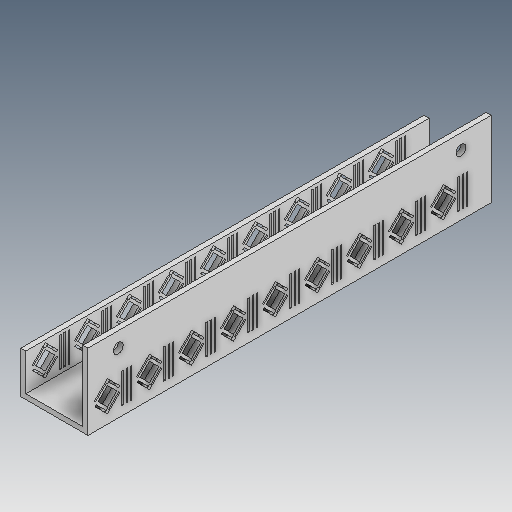
# Autodesk Inventor part: cable_basket
Saved by Autodesk Inventor 2027 (Build 310192060, 192F)
## iProperties
Created: 2026-07-28
Part Number: cable_basket
Material: Generic
Document SubType Name: Modeling
Designer: prest
Density: 1 g/cm^3
Appearance: Default
Author: prest
Autodesk Inventor part; units mm, degrees
ref_plane "YZ Plane" through (0, 0, 0) normal (1, 0, 0) x (0, 1, 0)
ref_plane "XZ Plane" through (0, 0, 0) normal (0, 1, 0) x (-1, 0, 0)
ref_plane "XY Plane" through (0, 0, 0) normal (0, 0, 1) x (1, 0, 0)
sketch "Sketch1" plane through (0, 0, 0) normal (0, 1, 0) x (-1, 0, 0)
  line L0 (65.1379, 125.1379) -> (25.1379, 125.1379)
  line L1 (25.1379, 125.1379) -> (25.1379, -114.8621)
  line L2 (25.1379, -114.8621) -> (65.1379, -114.8621)
  line L3 (65.1379, -114.8621) -> (65.1379, 125.1379)
  point P0 (0, 0)
  dimension "d0" = 240
  dimension "d1" = 40
  constraints: 8 end point, 2 parallel, 1 horizontal, 1 perpendicular
  measures "d0" distance of L2.end L0.start
  measures "d1" distance of L0.start L0.end
extrude "Extrusion1" add sketch "Sketch1" along normal blind 25
sketch "Sketch2" plane through (-65.1379, 0, 125.1379) normal (0, 0, 1) x (1, 0, 0)
  line L0 (0, 0) -> (0, 25) projected
  line L1 (0, 0) -> (40, 0) projected
  line L2 (40, 0) -> (40, 25) projected
  line L3 (3, 25) -> (3, 3)
  line L4 (3, 3) -> (37, 3)
  line L5 (37, 3) -> (37, 25)
  line L6 (3, 25) -> (37, 25)
  point P0 (65.1379, 0)
  dimension "d4" = 3
  constraints: 8 end point, 1 perpendicular, 2 other
  measures "d4" distance between parallel lines of L0 L3
extrude "Extrusion2" cut sketch "Sketch2" against normal through all
sketch "Sketch3" plane through (-65.1379, 0, -114.8621) normal (-1, 0, 0) x (0, 0, 1)
  line L0 (240, 3) -> (0, 3) projected
  line L1 (219.8357, 5.3002) -> (219.8357, 23)
  line L2 (219.8357, 23) -> (218.8357, 23)
  line L3 (218.8357, 23) -> (218.8357, 5.3002)
  line L4 (217.3357, 23) -> (216.3357, 23)
  line L5 (216.3357, 23) -> (216.3357, 5.3002)
  line L6 (217.3357, 5.3002) -> (217.3357, 23)
  line L7 (240, 0) -> (240, 25) projected
  line L8 (0, 25) -> (240, 25) projected
  line L9 (213.8357, 23) -> (214.8357, 23)
  line L10 (214.8357, 23) -> (214.8357, 5.3002)
  line L11 (213.8357, 5.3002) -> (213.8357, 23)
  line L12 (222.8357, 14.4178) -> (228.4178, 8.8357)
  line L13 (228.4178, 8.8357) -> (234, 14.4178)
  line L14 (234, 14.4178) -> (228.4178, 20)
  line L15 (228.4178, 20) -> (222.8357, 14.4178)
  line L16 (221.775, 15.4785) -> (227.3572, 21.0607)
  line L17 (229.4785, 21.0607) -> (235.4217, 15.1174)
  line L18 (235.0607, 13.3572) -> (229.4785, 7.775)
  line L19 (227.3572, 7.775) -> (221.775, 13.3572)
  line L20 (221.0679, 16.1856) -> (226.6501, 21.7678)
  line L21 (230.144, 21.8094) -> (236.1288, 15.8245)
  line L22 (226.6501, 7.0679) -> (221.0679, 12.6501)
  line L23 (235.7678, 12.6501) -> (230.1856, 7.0679)
  line L24 (221.0679, 16.1856) -> (221.775, 15.4785)
  line L25 (226.6501, 21.7678) -> (227.3572, 21.0607)
  line L26 (230.144, 21.8094) -> (229.4785, 21.0607)
  line L27 (236.1288, 15.8245) -> (235.4217, 15.1174)
  line L28 (235.0607, 13.3572) -> (235.7678, 12.6501)
  line L29 (226.6501, 7.0679) -> (227.3572, 7.775)
  line L30 (229.4785, 7.775) -> (230.1856, 7.0679)
  line L31 (221.0679, 12.6501) -> (221.775, 13.3572)
  line L32 (227.0036, 6.7144) -> (228.4178, 8.1286)
  line L33 (228.4178, 8.1286) -> (229.8321, 6.7144)
  line L34 (229.8321, 6.7144) -> (228.4178, 5.3002)
  line L35 (228.4178, 5.3002) -> (227.0036, 6.7144)
  line L36 (228.4178, 20.7071) -> (229.8321, 22.1213)
  line L37 (229.8321, 22.1213) -> (228.4178, 23.5355)
  line L38 (228.4178, 23.5355) -> (227.0036, 22.1213)
  line L39 (227.0036, 22.1213) -> (228.4178, 20.7071)
  line L40 (213.8357, 5.3002) -> (214.8357, 5.3002)
  line L41 (216.3357, 5.3002) -> (217.3357, 5.3002)
  line L42 (218.8357, 5.3002) -> (219.8357, 5.3002)
  line L43 (228.4178, 20) -> (228.4178, 8.8357) construction
  line L44 (222.8357, 14.4178) -> (234, 14.4178) construction
  point P0 (114.8621, 0)
  point P1 (216.8357, 23)
  point P2 (219.3357, 23)
  point P3 (214.3357, 23)
  point P4 (219.3357, 5.3002)
  dimension "d9" = 1
  dimension "d10" = 1
  dimension "d11" = 1.5
  dimension "d13" = 2
  dimension "d15" = 1
  dimension "d16" = 1.5
  dimension "d17" = 5
  dimension "d20" = 3
  dimension "d21" = 1.5
  dimension "d22" = 1.5
  dimension "d23" = 1
  dimension "d24" = 1
  dimension "d25" = 1
  dimension "d26" = 1
  dimension "d27" = 6
  dimension "d29" = 1.5
  dimension "d30" = 5.5822
  dimension "d31" = 0.5
  constraints: 84 end point, 24 perpendicular, 11 collinear, 6 horizontal, 5 vertical alignment, 4 horizontal alignment, 4 midpoint, 4 parallel, 2 point on line, 2 vertical
  measures "d9" distance of L1.end L2.end
  measures "d10" distance of L4.start L4.end
  measures "d11" distance between parallel lines of L3 L6
  measures "d13" distance from line of L8 point (216.836, 23)
  measures "d15" distance of L9.end L9.start
  measures "d16" distance of L4.end L9.end
  measures "d17" distance from line of L8 L14.end
  measures "d20" distance from line of L12.start L1
  measures "d21" distance between parallel lines of L15 L16
  measures "d22" distance between parallel lines of L17 L14
  measures "d23" distance between parallel lines of L16 L20
  measures "d24" distance between parallel lines of L17 L21
  measures "d25" distance between parallel lines of L19 L22
  measures "d26" distance between parallel lines of L18 L23
  measures "d27" distance from line of L7 L13.end
  measures "d29" distance between parallel lines of L12 L19
  measures "d30" horizontal distance of L12.end L13.end
  measures "d31" distance between parallel lines of L39 L25
extrude "Extrusion3" cut sketch "Sketch3" against normal through all
pattern_linear "Rectangular Pattern1" count 9 spacing 25 along (0, 0, -1) of "Extrusion3"
move faces "Move1" translate (0, 20, 0) faces at (-27.1379, 25, -34.8621)
sketch "Sketch5" plane through (-25.1379, 0, 125.1379) normal (1, 0, 0) x (0, 0, -1)
  line L0 (0, 0) -> (0, 45) projected
  line L1 (240, 3) -> (240, 45) projected
  line L2 (0, 45) -> (240, 45) projected
  point P0 (125.1379, 0)
  point P1 (18, 36)
  point P2 (222, 36)
  dimension "d40" = 204
  dimension "d41" = 18
  dimension "d43" = 9
  constraints: 1 horizontal alignment
  measures "d40" distance of point (222, 36) point (18, 36)
  measures "d41" distance from line of point (18, 36) L0
  measures "d43" distance from line of L2 point (222, 36)
hole "Hole1" at (-25.1379, 36, 107.1379) at (-25.1379, 36, -96.8621) direction (-1, 0, 0) diameter 6 depth 8
equation "\"d29\" = d21"
body "Solid1"
